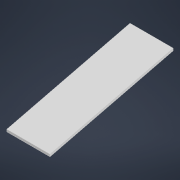
# Autodesk Inventor part: TorraumSchrägeUntenNEU
Saved by Autodesk Inventor 2021.4 (Build 254397000, 397)
## iProperties
Created: 2022-02-22
Part Number: TorraumSchrägeUntenNEU
Material: Generisch
Document SubType Name: Modeling
Designer: valen
Density: 1 g/cm^3
Appearance: Vorgabe
Author: valen
Autodesk Inventor part; units mm, degrees
ref_plane "YZ Plane" through (0, 0, 0) normal (1, 0, 0) x (0, 1, 0)
ref_plane "XZ Plane" through (0, 0, 0) normal (0, 1, 0) x (-1, 0, 0)
ref_plane "XY Plane" through (0, 0, 0) normal (0, 0, 1) x (1, 0, 0)
sketch "Skizze1" plane through (0, 0, 0) normal (1, 0, 0) x (0, 1, 0)
  line L0 (55.8816, -228) -> (0, 0)
  line L1 (0, 0) -> (4.1184, 0)
  line L2 (55.8816, -228) -> (60, -228)
  line L3 (60, -228) -> (4.1184, 0)
  line L4 (0, 0) -> (0, -228)
  line L5 (0, -228) -> (60, -228)
  dimension "d17" = 228
  dimension "d18" = 60
  dimension "d19" = 4
  constraints: 12 end point, 2 horizontal, 1 perpendicular, 1 vertical
  measures "d17" distance of L0.end L4.end
  measures "d18" distance of L4.end L2.end
  measures "d19" distance between parallel lines of L3 L0
extrude "Extrusion2" add sketch "Skizze1" along normal blind 80 contours L0 L1 L3 L2
